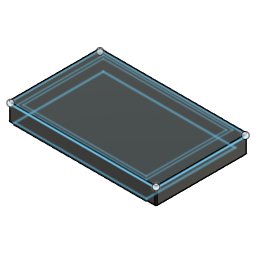
Removable base (Autodesk Fusion 360 design; units mm, degrees)
Autodesk Fusion 360 part; units mm, degrees
sketch "sketch 590" plane through (0, 0, -7.8648) normal (0, 0, -1) x (1, 0, 0)
  line L0 (62.9677, 34.6352) -> (62.9677, -50.3648)
  line L1 (62.9677, -50.3648) -> (-64.5323, -50.3648)
  line L2 (-64.5323, -50.3648) -> (-64.5323, 34.6352)
  line L3 (-64.5323, 34.6352) -> (62.9677, 34.6352)
  line L4 (74, 37.1352) -> (-69.252, 37.1352)
  arc A0 (-69.252, 37.1352) -> (-70.252, 36.1352) centre (-69.252, 36.1352) ccw
  line L5 (-70.252, 36.1352) -> (-70.252, -51.8648)
  arc A1 (-70.252, -51.8648) -> (-69.252, -52.8648) centre (-69.252, -51.8648) ccw
  line L6 (-69.252, -52.8648) -> (74, -52.8648)
  arc A2 (74, -52.8648) -> (75, -51.8648) centre (74, -51.8648) ccw
  line L7 (75, -51.8648) -> (75, 36.1352)
  arc A3 (75, 36.1352) -> (74, 37.1352) centre (74, 36.1352) ccw
extrude "Extrude1" add sketch "sketch 590" along normal blind 15.196
sketch "sketch 644" plane through (0, 0, -23.0608) normal (0, 0, -1) x (1, 0, 0)
  line L0 (-65.2823, -51.1148) -> (-65.2823, 35.3852)
  line L1 (-65.2823, 35.3852) -> (63.7177, 35.3852)
  line L2 (63.7177, 35.3852) -> (63.7177, -51.1148)
  line L3 (63.7177, -51.1148) -> (-65.2823, -51.1148)
  line L4 (-66.2823, -52.1148) -> (-66.2823, 36.3852)
  line L5 (64.7177, -52.1148) -> (-66.2823, -52.1148)
  line L6 (64.7177, 36.3852) -> (64.7177, -52.1148)
  line L7 (-66.2823, 36.3852) -> (64.7177, 36.3852)
extrude "Extrude2" add sketch "sketch 644" along normal blind 1.5
sketch "sketch 677" plane through (0, 15.7296, -7.8648) normal (0, 0, 1) x (1, 0, 0)
  line L0 (59.9677, 31.6352) -> (59.9677, -47.3648)
  line L1 (59.9677, -47.3648) -> (-61.5323, -47.3648)
  line L2 (-61.5323, -47.3648) -> (-61.5323, 31.6352)
  line L3 (-61.5323, 31.6352) -> (59.9677, 31.6352)
  arc A0 (-70.252, -51.8648) -> (-69.252, -52.8648) centre (-69.252, -51.8648) ccw
  line L4 (-69.252, -52.8648) -> (74, -52.8648)
  arc A1 (74, -52.8648) -> (75, -51.8648) centre (74, -51.8648) ccw
  line L5 (75, -51.8648) -> (75, 36.1352)
  arc A2 (75, 36.1352) -> (74, 37.1352) centre (74, 36.1352) ccw
  line L6 (74, 37.1352) -> (-69.252, 37.1352)
  arc A3 (-69.252, 37.1352) -> (-70.252, 36.1352) centre (-69.252, 36.1352) ccw
  line L7 (-70.252, 36.1352) -> (-70.252, -51.8648)
extrude "Extrude3" add sketch "sketch 677" along normal blind 1.5
extrude "Extrude4" add 1 faces at (19.4677, -31.6352, -7.3648) along direction (0, 1, 0) blind 79
extrude "Extrude5" add 1 faces at (-21.5013, -7.1352, -6.3648) along direction (0, 0, 1) blind 0.304
